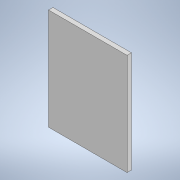
# Autodesk Inventor part: back_plate
Saved by Autodesk Inventor 2022.1 (Build 261234020, 234B)
## iProperties
Created: 2022-01-26
Part Number: back_plate
Material: Generic
Document SubType Name: Modeling
Designer: logic
Density: 1 g/cm^3
Appearance: Default
Author: logic
Autodesk Inventor part; units mm, degrees
ref_plane "YZ Plane" through (0, 0, 0) normal (1, 0, 0) x (0, 1, 0)
ref_plane "XZ Plane" through (0, 0, 0) normal (0, 1, 0) x (-1, 0, 0)
ref_plane "XY Plane" through (0, 0, 0) normal (0, 0, 1) x (1, 0, 0)
sketch "Sketch1" plane through (0, 0, 0) normal (0, 0, 1) x (1, 0, 0)
  line L0 (44.5, 57.5) -> (-44.5, 57.5)
  line L1 (-44.5, 57.5) -> (-44.5, -57.5)
  line L2 (-44.5, -57.5) -> (44.5, -57.5)
  line L3 (44.5, -57.5) -> (44.5, 57.5)
  point P0 (0, 0)
  dimension "d0" = 89
  dimension "d3" = 115
  dimension "d4" = 57.5
  dimension "d5" = 44.5
  constraints: 8 end point, 2 parallel, 1 horizontal, 1 perpendicular
  measures "d0" distance of L1.end L2.end
  measures "d3" distance of L0.end L1.end
  measures "d4" vertical distance of L1.end point (0, 0)
  measures "d5" horizontal distance of L1.end point (0, 0)
extrude "Extrusion1" add sketch "Sketch1" along normal blind 5
equation "\"d4\" = 0.5 * d3"
equation "\"d5\" = 0.5 * d0"
body "Solid1"
